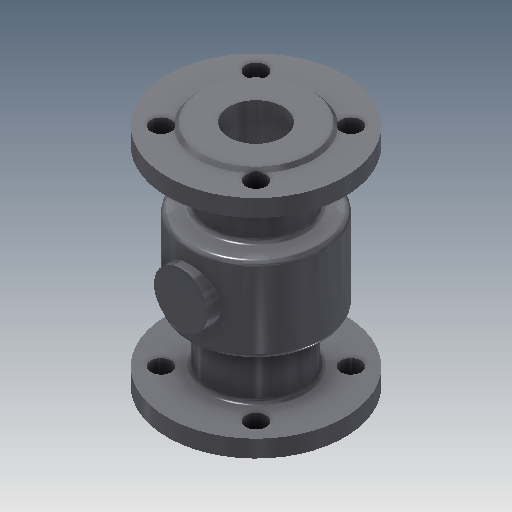
# Autodesk Inventor part: Flanged Ball Valve
Saved by Autodesk Inventor 2019.1 (Build 231200000, 200)
## iProperties
Created: 2002-04-25
Part Number: Flanged Ball Valve
Material: Cast Iron
Document SubType Name: Modeling
Designer: D.Ali
Description: Flanged Ball Valve
Standard: BS4504
Standard Revision: 1
Manufacturer: Datech
Standards Organization: Custom
Language: ENG
Categories: <domain><piping version="1" type="fitting"><fitting><connection index="1" flipDirection="False"><display>Connection1</display><NS><bound-to>ND</bound-to></NS><Female>False</Female><EndTreatment>Flanged</EndTreatment><Fixed>False</Fixed><MaxEngagement> 0</MaxEngagement><MinEngagement> 0</MinEngagement></connection></fitting></piping></domain>
Density: 7.05 g/cm^3
Appearance: Metal-Steel (Polished)
Stock Number: NA
Mass: 12920 g
Surface Area: 1930.88 cm^2
Volume: 1832.62 cm^3
NAME: PIPING: BS4504 Flange PN16
DATA: <meta><inlinegroups number="0" deflen="0"></inlinegroups><connections number="1"></connections><angles></angles></meta>
Control State: 0
Master: False
Checked Out: False
Shininess: 41.0
Angle Display Precision: 2
Document Length Units: 11269
Document Angle Units: 11279
Document Time Units: 11290
Document Mass Units: 11283
Document Length Units Precision: 3
Document Angle Units Precision: 2
Face_face: 229.000 mm
NB: 100.000 mm
PCD: 180.000 mm
FlangeOD: 220.000 mm
Holenum: 8.000 ul
FlangefaceOD: 156.000 mm
Holedia: 19.000 mm
Flangethk: 16.000 mm
PipeOD: 110.000 mm
Flangefacethk: 3.000 mm
Density: 0.0
Volumn: 0.0
Area: 0.0
PropertySet Name: Model Information
Author: Demir Ali
Title: Purchased Part
Revision Number: A
Autodesk Inventor part; units mm, degrees
ref_plane "YZ Plane" through (0, 0, 0) normal (1, 0, 0) x (0, 1, 0)
ref_plane "XZ Plane" through (0, 0, 0) normal (0, 1, 0) x (-1, 0, 0)
ref_plane "XY Plane" through (0, 0, 0) normal (0, 0, 1) x (1, 0, 0)
sketch "Sketch27" plane through (0, 0, 0) normal (0, 1, 0) x (-1, 0, 0)
  circle A0 centre (0, 0) radius 82.5
  dimension "d21" = 165
  constraints: 1 centre point, 1 coincident
  measures "d21" diameter of A0
extrude "Extrusion20" add sketch "Sketch27" against normal blind 16
sketch "Sketch55" plane through (0, -16, 0) normal (0, -1, 0) x (1, 0, 0)
  circle A0 centre (0, 0) radius 82.5 projected
  circle A1 centre (0, 0) radius 51
  dimension "d275" = 102
  constraints: 1 centre point, 1 coincident
  measures "d275" diameter of A1
extrude "Extrusion39" add sketch "Sketch55" along normal blind 3 contours A1
chamfer "Chamfer8" distance 3 angle 45 1 edges at (-51, -16, 0)
sketch "Sketch29" plane through (0, 0, 0) normal (0, 1, 0) x (1, 0, 0)
  circle A0 centre (0, 0) radius 62.5
  circle A1 centre (0, 0) radius 62.5 construction
  line L0 (0, 0) -> (-44.1942, -44.1942) construction
  circle A2 centre (0, 0) radius 82.5 projected
  line L1 (0, 99) -> (0, -132) projected
  dimension "d29" = 125
  dimension "d30" = 45
  constraints: 3 coincident, 2 end point, 6 other
  measures "d30" angle of L1 L0
hole "Hole2" at (-44.1942, 0, 44.1942) direction (0, -1, 0) diameter 19 end through all
pattern_circular "Circular Pattern2" count 4 over 360 about axis through (0, 0, 0) along (0, -1, 0) of "Hole2"
ref_plane "Work Plane11" through (0, 89, 0) normal (0, -1, 0) x (1, 0, 0)
mirror "Mirror5" about plane through (0, 89, 0) normal (0, -1, 0) of "Extrusion20", "Extrusion39", "Chamfer8", "Hole2", "Circular Pattern2"
sketch "Sketch57" plane through (0, 0, 0) normal (0, 1, 0) x (1, 0, 0)
  circle A0 centre (0, 0) radius 82.5 projected
  circle A1 centre (0, 0) radius 42.5
  dimension "d289" = 85
  constraints: 1 centre point, 1 coincident
  measures "d289" diameter of A1
extrude "Extrusion40" add sketch "Sketch57" along normal up to next contours A1
sketch "Sketch58" plane through (0, 89, 0) normal (0, -1, 0) x (1, 0, 0)
  circle A0 centre (0, 0) radius 42.5 projected
  circle A1 centre (0, 0) radius 62.5
  dimension "d292" = 125
  constraints: 1 centre point, 1 coincident
  measures "d292" diameter of A1
extrude "Extrusion41" add sketch "Sketch58" along normal mid plane 80 contours A0 | A1
fillet "Fillet56" radius 5 6 edges at (-42.5, 129, 0) (-62.5, 129, 0) (-42.5, 49, 0) (-62.5, 49, 0) (-42.5, 0, 0) (-42.5, 178, 0)
ref_plane "Work Plane12" through (0, 89, 62.5) normal (0, 0, 1) x (1, 0, 0)
sketch "Sketch59" plane through (0, 89, 62.5) normal (0, 0, 1) x (1, 0, 0)
  line L0 (0, -129.6) -> (0, 172.8) projected
  line L1 (51, -108) -> (-51, -108) projected
  circle A0 centre (0, 0) radius 25
  line L2 (132, 0) -> (-99, 0) projected
  dimension "d297" = 50
  constraints: 2 point on line, 1 centre point
  measures "d297" diameter of A0
extrude "Extrusion42" add sketch "Sketch59" along normal mid plane 15
sketch "Sketch56" plane through (0, -19, 0) normal (0, -1, 0) x (1, 0, 0)
  circle A0 centre (0, 0) radius 51 projected
hole "Hole6" at (0, -19, 0) direction (0, 1, 0) diameter 50 end through all
sketch "Sketch60" plane through (0, 84.0068, 13.3927) normal (1, 0, 0) x (0, 0, -1)
  line L0 (-59.69, -7.4528) -> (-59.69, 24.2972)
  arc A0 (-59.69, 24.2972) -> (-61.8522, 29.6148) centre (-67.31, 24.2972) ccw
  line L1 (-61.8522, 29.6148) -> (-84.0089, 52.3556)
  arc A1 (-85.09, 55.0144) -> (-84.0089, 52.3556) centre (-81.28, 55.0144) ccw
  line L2 (-85.09, 55.0144) -> (-85.09, 170.3472)
  line L3 (-85.09, 170.3472) -> (-88.9, 170.3472)
  line L4 (-88.9, 170.3472) -> (-88.9, 55.0144)
  arc A2 (-88.9, 55.0144) -> (-86.7378, 49.6968) centre (-81.28, 55.0144) ccw
  line L5 (-86.7378, 49.6968) -> (-64.5811, 26.956)
  arc A3 (-63.5, 24.2972) -> (-64.5811, 26.956) centre (-67.31, 24.2972) ccw
  line L6 (-63.5, 24.2972) -> (-63.5, -7.4528)
  line L7 (-63.5, -7.4528) -> (-59.69, -7.4528)
  line L8 (0, -18.034) -> (0, 124.206)
  line L9 (-28.0662, 4.9932) -> (-56.6073, 4.9932)
  line L10 (-56.6073, -20.0068) -> (-56.6073, 29.9932) projected
  dimension "d306" = 3.81
  dimension "d307" = 3.81
  dimension "d308" = 3.81
  dimension "d304" = 177.8
  dimension "d311" = 31.75
  dimension "d309" = 31.75
  dimension "d305" = 25.4
  dimension "d310" = 59.69
  dimension "d303" = 12.446
  dimension "d321" = 16
  dimension "d324" = 20
  constraints: 12 end point, 2 coincident, 1 centre point, 11 other
  measures "d324" distance between parallel lines of L1 L4
sketch "Sketch62" plane through (0, 0, 0) normal (1, 0, 0) x (0, 1, 0)
  line L0 (89, 76.8927) -> (79, 76.8927) projected
  line L1 (79, 84.8927) -> (89, 84.8927) projected
  line L2 (73.6393, 84.8927) -> (73.6393, 82.8927)
  line L3 (73.6393, 82.8927) -> (82.6108, 84.8927)
  line L4 (73.6393, 76.8927) -> (73.6393, 78.8927)
  line L5 (73.6393, 78.8927) -> (82.6108, 76.8927)
  line L6 (89, 157.7306) -> (89, -100.9793) projected
  line L7 (73.6393, 84.8927) -> (82.6108, 84.8927)
  line L8 (73.6393, 76.8927) -> (82.6108, 76.8927)
  dimension "d330" = 2
  constraints: 12 end point, 2 equal length, 2 perpendicular, 2 point on line, 2 vertical alignment, 1 collinear
  measures "d330" distance of L2.start L2.end
equation "\"NB\" = 50"
equation "\"PipeOD\" = 60.325"
equation "\"FlangeOD\" = 165"
equation "\"FlangefaceOD\" = 102"
equation "\"Holedia\" = 19"
equation "\"Holenum\" = 4"
equation "\"PCD\" = 125"
equation "\"Flangethk\" = 16"
equation "\"Flangefacethk\" = 3"
body "Solid1"
